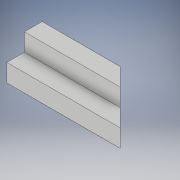
# Autodesk Inventor part: 8.3 part 1
Saved by Autodesk Inventor 2017.3 (Build 213256000, 256)
## iProperties
Created: 2017-05-01
Part Number: 8.3 part 1
Material: Generic
Document SubType Name: Modeling
Designer: rbibb
Density: 1 g/cm^3
Appearance: Default
Author: rbibb
Autodesk Inventor part; units mm, degrees
ref_plane "YZ Plane" through (0, 0, 0) normal (1, 0, 0) x (0, 1, 0)
ref_plane "XZ Plane" through (0, 0, 0) normal (0, 1, 0) x (-1, 0, 0)
sketch "Sketch1" plane through (0, 0, 0) normal (1, 0, 0) x (0, 1, 0)
  line L0 (-181.551, 47.1304) -> (-181.551, -16.3696)
  line L1 (8.949, -16.3696) -> (8.949, 47.1304)
  line L2 (-54.5587, 110.3897) -> (-118.0587, 110.3897)
  line L3 (-118.0587, -80.1103) -> (-54.5587, -80.1103)
  line L4 (8.949, 47.1304) -> (-54.5587, 47.1304)
  line L5 (-118.0587, 47.1304) -> (-181.551, 47.1304)
  line L6 (-54.5587, -80.1103) -> (-54.5587, -16.3696)
  line L7 (-54.5587, 47.1304) -> (-54.5587, 110.3897)
  line L8 (-181.551, -16.3696) -> (-118.0587, -16.3696)
  line L9 (-54.5587, -16.3696) -> (8.949, -16.3696)
  line L10 (-118.0587, 110.3897) -> (-118.0587, 47.1304)
  line L11 (-118.0587, -16.3696) -> (-118.0587, -80.1103)
  point P0 (0, 0)
  dimension "d0" = 190.5
  dimension "d1" = 63.5
  dimension "d3" = 63.5
  dimension "d4" = 190.5
  constraints: 24 end point, 10 parallel, 8 perpendicular, 3 horizontal
  measures "d0" distance of L1.start L0.end
  measures "d1" distance of L0.start L0.end
  measures "d3" distance of L3.end L3.start
  measures "d4" distance of L2.end L3.start
extrude "Extrusion1" add sketch "Sketch1" along normal blind 406.4
ref_plane "Work Plane1" through (406.4, 0, 110.3897) normal (0.7071, 0, -0.7071) x (0, 1, 0)
sketch "Sketch2" plane through (406.4, 0, 0) normal (1, 0, 0) x (0, 0, -1)
  line L0 (-47.1304, 8.949) -> (16.3696, 8.949) projected
  line L1 (-48.288, 8.949) -> (16.3696, 8.949)
  line L2 (16.3696, -54.5587) -> (16.3696, 8.949) projected
  line L3 (16.3696, 8.949) -> (16.3696, -54.5587)
  line L4 (16.3696, -54.5587) -> (80.1103, -54.5587)
  line L5 (16.3696, -118.0587) -> (80.1103, -118.0587) projected
  line L6 (80.1103, -54.5587) -> (80.1103, -118.0587)
  line L7 (80.1103, -118.0587) -> (16.3696, -118.0587)
  line L8 (16.3696, -181.551) -> (-47.1304, -181.551) projected
  line L9 (16.3696, -118.0587) -> (16.3696, -181.551)
  line L10 (16.3696, -181.551) -> (-47.1304, -181.551)
  line L11 (-47.1304, -181.551) -> (-47.1304, -118.0587) projected
  line L12 (-47.1304, -181.551) -> (-47.1304, -118.0587)
  line L13 (-47.1304, -118.0587) -> (-110.3897, -118.0587) projected
  line L14 (-47.1304, -118.0587) -> (-110.3897, -118.0587)
  line L15 (-110.3897, -118.0587) -> (-110.3897, -54.5587)
  line L16 (-110.3897, -54.5587) -> (-47.1304, -54.5587)
  line L17 (-47.1304, -54.5587) -> (-47.1304, 8.949) projected
  line L18 (-47.1304, -54.5587) -> (-47.1304, 8.949)
  line L19 (-47.1304, -54.5587) -> (-47.1304, 8.949)
  point P0 (0, 0)
  constraints: 26 end point, 7 perpendicular, 4 collinear, 2 vertical, 1 point on line
extrude "Extrusion2" cut sketch "Sketch2" against normal up to surface surface through (406.4, 0, 110.3897) normal (0.7071, 0, -0.7071)
body "Solid1"
